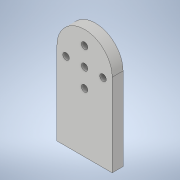
# Autodesk Inventor part: Tilt_Camera_Side_Plate
Saved by Autodesk Inventor 2022 (Build 260153000, 153)
## iProperties
Created: 2019-12-31
Part Number: Tilt_Camera_Side_Plate
Material: Generic
Document SubType Name: Modeling
Designer: KappaCat
Density: 1 g/cm^3
Appearance: Default
Author: KappaCat
Autodesk Inventor part; units mm, degrees
ref_plane "YZ Plane" through (0, 0, 0) normal (1, 0, 0) x (0, 1, 0)
ref_plane "XZ Plane" through (0, 0, 0) normal (0, 1, 0) x (-1, 0, 0)
ref_plane "XY Plane" through (0, 0, 0) normal (0, 0, 1) x (1, 0, 0)
sketch "Sketch1" plane through (0, 0, 0) normal (0, 0, 1) x (1, 0, 0)
  line L0 (9.2688, 23.2165) -> (-16.1312, 23.2165)
  line L1 (-16.1312, 23.2165) -> (-16.1312, -27.5835)
  line L2 (-16.1312, -27.5835) -> (9.2688, -27.5835)
  line L3 (9.2688, -27.5835) -> (9.2688, 23.2165)
  point P0 (0, 0)
  dimension "d0" = 25.4
  dimension "d1" = 50.8
  constraints: 8 end point, 2 parallel, 1 horizontal, 1 perpendicular
  measures "d0" distance of L0.start L0.end
  measures "d1" distance of L2.end L0.start
extrude "Extrusion1" add sketch "Sketch1" along normal blind 5
sketch "Sketch2" plane through (0, 0, 5) normal (0, 0, 1) x (1, 0, 0)
  circle A0 centre (-3.4312, 8.2165) radius 12.3 construction
  circle A1 centre (-3.4312, 8.2165) radius 8.5 construction
  circle A2 centre (-11.9312, 8.2165) radius 1.5
  circle A3 centre (-3.4312, 8.2165) radius 1.5
  circle A4 centre (-3.4312, -0.2835) radius 1.5
  circle A5 centre (5.0688, 8.2165) radius 1.5
  circle A6 centre (-3.4312, 16.7165) radius 1.5
  line L0 (9.2688, 23.2165) -> (-16.1312, 23.2165) projected
  point P0 (0, 0)
  point P1 (-3.4312, 23.2165)
  dimension "d5" = 17
  dimension "d4" = 24.6
  dimension "d6" = 3
  dimension "d7" = 3
  dimension "d10" = 360
  dimension "d12" = 15
  constraints: 6 centre point, 2 coincident, 2 vertical alignment, 1 horizontal alignment, 1 midpoint, 11 other
  measures "d4" diameter of A0
  measures "d6" diameter of A2
  measures "d7" diameter of A3
  measures "d12" distance of point (-3.431, 23.216) A0.centre
extrude "Extrusion2" cut sketch "Sketch2" against normal up to next
sketch "Sketch3" plane through (-16.1312, -27.5835, 0) normal (-1, 0, 0) x (0, 0, 1)
  line L0 (0, 0) -> (5, 0) projected
  point P0 (0, 27.5835)
  point P1 (2.5, 2.5)
  point P2 (2.5, 0)
  dimension "d15" = 2.5
  constraints: 1 midpoint, 1 vertical alignment
  measures "d15" distance from line of L0 point (2.5, 2.5)
hole "Hole1" at (-16.1312, -25.0835, 2.5) direction (1, 0, 0) diameter 2.46 depth 13.6906 tip angle 118
full round fillet "Fillet1" first side at (-16.1312, 7.5235, 2.4506) centre faces at (0.8021, 23.2165, 3.3333) second side at (9.2688, -10.6502, 1.6667)
body "Solid1"
